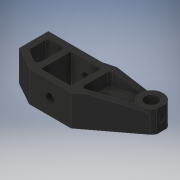
# Autodesk Inventor part: Y Foot Left
Saved by Autodesk Inventor 2019.4 (Build 234330000, 330)
## iProperties
Created: 2018-06-15
Part Number: Y Foot Left
Material: ABS Plastic
Document SubType Name: Modeling
Designer: Richard
Density: 1.06 g/cm^3
Appearance: Rubber - Black
Author: Richard
Autodesk Inventor part; units mm, degrees
ref_plane "YZ Plane" through (0, 0, 0) normal (1, 0, 0) x (0, 1, 0)
ref_plane "XZ Plane" through (0, 0, 0) normal (0, 1, 0) x (-1, 0, 0)
ref_plane "XY Plane" through (0, 0, 0) normal (0, 0, 1) x (1, 0, 0)
sketch "Sketch1" plane through (0, 0, 0) normal (0, 1, 0) x (-1, 0, 0)
  line L0 (38.625, 18.6875) -> (-38.625, 18.6875)
  line L1 (-38.625, 18.6875) -> (-38.625, -18.6875)
  line L2 (-38.625, -18.6875) -> (38.625, -18.6875)
  line L3 (38.625, -18.6875) -> (38.625, 18.6875)
  line L4 (38.625, 18.6875) -> (-38.625, -18.6875) construction
  line L5 (-38.625, 18.6875) -> (38.625, -18.6875) construction
  point P0 (0, 0)
  dimension "d0" = 77.25
  dimension "d2" = 37.375
  constraints: 12 end point, 2 midpoint, 2 parallel, 1 horizontal, 1 perpendicular
  measures "d0" distance of L2.end L1.end
  measures "d2" distance of L0.end L1.end
extrude "Extrusion1" add sketch "Sketch1" along normal mid plane 21
sketch "Sketch2" plane through (0, 10.5, 0) normal (0, 1, 0) x (1, 0, 0)
  line L0 (-19, 6.0625) -> (1.75, 6.0625)
  line L1 (1.75, 6.0625) -> (1.75, -14.6875)
  line L2 (1.75, -14.6875) -> (-19, -14.6875)
  line L3 (-19, -14.6875) -> (-19, 6.0625)
  line L4 (-19, 6.0625) -> (1.75, -14.6875) construction
  line L5 (1.75, 6.0625) -> (-19, -14.6875) construction
  line L6 (-38.625, -18.6875) -> (38.625, -18.6875) projected
  line L7 (-38.625, 18.6875) -> (-38.625, -18.6875) projected
  line L8 (-38.625, 10.0625) -> (-1.8672, 10.0625)
  line L9 (-1.8672, 10.0625) -> (29.3044, 18.4149)
  arc A0 (36.196, 4.3033) -> (29.3044, 18.4149) centre (31.375, 10.6875) ccw
  line L10 (38.625, 18.6875) -> (-38.625, 18.6875) projected
  line L11 (36.196, 4.3033) -> (5.75, -18.6875)
  line L12 (-38.625, -9.9375) -> (-23, -18.6875)
  arc A1 (29.3044, 18.4149) -> (36.196, 4.3033) centre (31.375, 10.6875) ccw construction
  circle A2 centre (9.875, -0.3125) radius 3.9
  circle A3 centre (31.375, 10.6875) radius 4.375
  point P0 (0, 0)
  point P1 (-8.625, -4.3125)
  dimension "d5" = 20.75
  dimension "d6" = 20.75
  dimension "d7" = 4
  dimension "d8" = 19.625
  dimension "d9" = 28.75
  dimension "d10" = 16
  dimension "d11" = 70
  dimension "d12" = 44.375
  dimension "d13" = 165
  dimension "d14" = 15.625
  dimension "d15" = 8.75
  dimension "d18" = 7.8
  dimension "d19" = 18.375
  dimension "d20" = 48.5
  dimension "d21" = 8.75
  constraints: 20 end point, 4 centre point, 4 point on circle, 4 point on line, 3 tangent, 2 horizontal, 2 midpoint, 2 parallel, 1 coincident, 1 perpendicular
  measures "d5" distance of L0.start L0.end
  measures "d6" distance of L2.end L0.start
  measures "d7" distance between parallel lines of L6 L2
  measures "d8" distance between parallel lines of L7 L3
  measures "d9" distance between parallel lines of L6 L8
  measures "d10" diameter of A0
  measures "d11" distance from line of L7 A0.centre
  measures "d12" distance from line of L7 L11.end
  measures "d13" angle of L8 L9
  measures "d14" distance from line of L12.end L7
  measures "d15" distance from line of L12.start L6
  measures "d18" diameter of A2
  measures "d19" distance from line of L6 A2.centre
  measures "d20" distance from line of L7 A2.centre
  measures "d21" diameter of A3
extrude "Extrusion2" cut sketch "Sketch2" against normal blind 23.75 contours L12 L7 L8 L9 A0 L11 L6 keep common part
sketch "Sketch3" plane through (0, 10.5, 0) normal (0, 1, 0) x (1, 0, 0)
  line L0 (-23, 6.0625) -> (-34.625, 6.0625)
  line L1 (-34.625, 6.0625) -> (-34.625, -7.593)
  line L2 (-34.625, -7.593) -> (-23, -14.103)
  line L3 (-23, -14.103) -> (-23, 6.0625)
  line L4 (-19, 6.0625) -> (-19, -14.6875) projected
  line L5 (-38.625, 10.0625) -> (-1.8672, 10.0625) projected
  line L6 (-38.625, 10.0625) -> (-38.625, -9.9375) projected
  line L7 (-23, -18.6875) -> (-38.625, -9.9375) projected
  point P0 (0, 0)
  dimension "d22" = 4
  dimension "d23" = 4
  dimension "d24" = 4
  dimension "d25" = 4
  constraints: 8 end point, 2 parallel, 1 horizontal, 1 perpendicular
  measures "d22" distance between parallel lines of L4 L3
  measures "d23" distance between parallel lines of L5 L0
  measures "d24" distance between parallel lines of L6 L1
  measures "d25" distance between parallel lines of L7 L2
extrude "Extrusion3" cut sketch "Sketch3" against normal blind 17
sketch "Sketch4" plane through (0, 10.5, 0) normal (0, 1, 0) x (1, 0, 0)
  line L0 (5.75, -13.6752) -> (5.75, 7.9624)
  line L1 (5.75, 7.9624) -> (23.2324, 12.6468)
  arc A0 (23.2324, 12.6468) -> (27.9136, 3.0613) centre (31.375, 10.6875) ccw
  line L2 (27.9136, 3.0613) -> (5.75, -13.6752)
  circle A1 centre (31.375, 10.6875) radius 4.375 projected
  line L3 (-1.8672, 10.0625) -> (29.3044, 18.4149) projected
  line L4 (36.196, 4.3033) -> (5.75, -18.6875) projected
  line L5 (1.75, -14.6875) -> (1.75, 6.0625) projected
  point P0 (0, 0)
  dimension "d28" = 4
  dimension "d29" = 4
  dimension "d30" = 4
  dimension "d31" = 4
  constraints: 6 end point, 2 parallel, 2 point on circle, 1 centre point, 1 concentric, 1 vertical
  measures "d28" radial gap between concentric circles of A1 A0
  measures "d29" distance between parallel lines of L3 L1
  measures "d30" distance between parallel lines of L4 L2
  measures "d31" distance between parallel lines of L5 L0
extrude "Extrusion4" cut sketch "Sketch4" against normal blind 9 contours L0 L1 A0 L2
fillet "Fillet1" radius 2 8 edges at (-34.625, 2, -6.0625) (-23, 2, -6.0625) (-34.625, 2, 7.593) (-23, 2, 14.103) (5.75, 6, 13.6752) (27.9136, 6, -3.0613) (5.75, 6, -7.9624) (23.2324, 6, -12.6468)
ref_plane "Work Plane1" through (7.2324, 10.5, -8.3596) normal (-0.8754261, 0.4226183, 0.2345697) x (0.258819, 0, 0.9659258)
sketch "Sketch5" plane through (7.2324, 10.5, -8.3596) normal (-0.8754261, 0.4226183, 0.2345697) x (0.258819, 0, 0.9659258)
  line L0 (-4, -3.5283) -> (-4, 10.1101) projected
  line L1 (0, 0) -> (0, 5.8077) projected
  line L2 (0, 0) -> (-4, 0)
  line L3 (-4, 0) -> (-4, 17.443)
  line L4 (-4, 17.443) -> (0, 17.443)
  line L5 (0, 17.443) -> (0, 0)
  point P0 (6.2029, -13.383)
  constraints: 8 end point, 2 parallel, 1 collinear, 1 horizontal, 1 perpendicular
extrude "Extrusion5" cut sketch "Sketch5" against normal blind 98.5
ref_plane "Work Plane2" through (8.9552, 10.5, 11.2548) normal (-0.770837, 0.258819, 0.5820851) x (-0.6026188, 0, -0.7980292)
sketch "Sketch6" plane through (8.9552, 10.5, 11.2548) normal (-0.770837, 0.258819, 0.5820851) x (-0.6026188, 0, -0.7980292)
  line L0 (-4, -8.053) -> (-4, 1.8213) projected
  line L1 (0, -5.4181) -> (0, 0) projected
  line L2 (0, 0) -> (-4, 0)
  line L3 (-4, 0) -> (-4, -11.4491)
  line L4 (-4, -11.4491) -> (0, -11.4491)
  line L5 (0, -11.4491) -> (0, 0)
  point P0 (14.3782, 10.2365)
  constraints: 8 end point, 2 parallel, 1 collinear, 1 horizontal, 1 perpendicular
extrude "Extrusion6" cut sketch "Sketch6" against normal blind 98.5
sketch "Sketch7" plane through (0, 10.5, 0) normal (0, 1, 0) x (1, 0, 0)
  line L0 (25.6612, 1.3605) -> (32.3712, 6.4274) projected
  arc A0 (28.6279, 14.0925) -> (32.3712, 6.4274) centre (31.375, 10.6875) ccw projected
  line L1 (28.6279, 14.0925) -> (20.5062, 11.9163) projected
  arc A1 (23.0192, 10.12) -> (20.5062, 11.9163) centre (21.0238, 9.9845) ccw projected
  arc A2 (23.0192, 10.12) -> (25.7898, 4.4468) centre (31.375, 10.6875) ccw projected
  arc A3 (25.6612, 1.3605) -> (25.7898, 4.4468) centre (24.456, 2.9565) ccw projected
  line L2 (35.1997, 8.5633) -> (38.625, 11.1499) projected
  line L3 (38.625, 11.1499) -> (38.625, 14.0694) projected
  arc A4 (38.625, 14.0694) -> (37.0319, 16.3444) centre (31.375, 10.6875) ccw projected
  line L4 (37.0319, 16.3444) -> (32.0515, 15.0099) projected
  arc A5 (35.1997, 8.5633) -> (32.0515, 15.0099) centre (31.375, 10.6875) ccw projected
  point P0 (0, 0)
extrude "Extrusion7" cut sketch "Sketch7" against normal up to surface (9 mm away)
sketch "Sketch8" plane through (0, -10.5, 0) normal (0, -1, 0) x (1, 0, 0)
  arc A0 (29.3044, -18.4149) -> (38.625, -14.0694) centre (31.375, -10.6875) ccw projected
  circle A1 centre (31.375, -10.6875) radius 4.375 projected
  arc A2 (38.625, -7.3056) -> (36.196, -4.3033) centre (31.375, -10.6875) ccw projected
  line L0 (38.625, -14.0694) -> (38.625, -7.3056) projected
  line L1 (36.196, -4.3033) -> (11.3657, 14.4469) projected
  arc A3 (36.196, -4.3033) -> (29.3044, -18.4149) centre (31.375, -10.6875) ccw
  point P0 (0, 0)
  constraints: 2 point on circle, 1 centre point, 1 concentric
extrude "Extrusion8" add sketch "Sketch8" against normal blind 15
fillet "Fillet2" radius 2 2 edges at (28.2566, 2.7597, -3.3203) (23.6476, 2.0377, -12.7581)
sketch "Sketch9" plane through (38.625, -10.5, -7.3056) normal (1, 0, 0) x (0, 0, -1)
  line L0 (0, 0) -> (0, 15) projected
  line L1 (6.7639, 0) -> (0, 0) projected
  line L2 (6.7639, 15) -> (6.7639, 0) projected
  line L3 (0, 15) -> (6.7639, 15) projected
  point P0 (-7.3056, 10.5)
  point P1 (3.3819, 7.5)
  point P2 (3.3819, 15)
  point P3 (6.7639, 7.5)
  constraints: 2 midpoint, 1 horizontal alignment, 1 vertical alignment
hole "Hole1" at (38.625, -3, -10.6875) direction (-1, 0, 0) diameter 5.2 end up to face face through (31.375, 10.5, -10.6875) facing (0, -1, 0) round with radius 4.375 far side no start extended yes
sketch "Sketch10" plane through (-1.8672, 10.5, -10.0625) normal (0, 0, -1) x (-1, 0, 0)
  line L0 (-3.6172, -21) -> (17.1328, -21) projected
  line L1 (17.1328, 0) -> (17.1328, -21) projected
  line L2 (17.1328, 0) -> (-3.6172, 0) projected
  line L3 (-3.6172, 0) -> (-3.6172, -21) projected
  point P0 (-1.8672, -10.5)
  point P1 (6.7578, -10.5)
  point P2 (6.7578, 0)
  point P3 (17.1328, -10.5)
  constraints: 2 midpoint, 1 horizontal alignment, 1 vertical alignment
hole "Hole2" at (-8.625, 0, -10.0625) direction (0, 0, 1) diameter 6 end through all start extended yes
equation "\"d6\" = d5"
equation "\"d23\" = d22"
equation "\"d24\" = d23"
equation "\"d25\" = d24"
body "Solid1"
